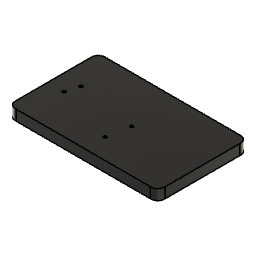
Modelo_Mesa_Optica (Autodesk Fusion 360 design; units mm, degrees)
Autodesk Fusion 360 part; units mm, degrees
sketch "Boceto1" plane through (0, 0, 0) normal (0, 0, 1) x (1, 0, 0)
  line L0 (-149.7985, 59.453) -> (50.2015, 59.453)
  line L1 (50.2015, 59.453) -> (50.2015, -60.547)
  line L2 (50.2015, -60.547) -> (-149.7985, -60.547)
  line L3 (-149.7985, -60.547) -> (-149.7985, 59.453)
  dimension "d22" = 120
  dimension "d23" = 200
  constraint horizontal L0
  constraint vertical L1
  constraint horizontal L2
  constraint vertical L3
  measures "d22" distance of L0.start L2.end
  measures "d23" distance of L1.end L2.end
extrude "Extruir1" add sketch "Boceto1" along normal blind 14
sketch "Boceto2" plane through (0, 0, 14) normal (0, 0, 1) x (-1, 0, 0)
  line L0 (20.6762, 30) -> (45, 30) construction
  line L1 (149.7985, 60.547) -> (-50.2015, 60.547)
  line L2 (-50.2015, 60.547) -> (-50.2015, -59.453)
  line L3 (-50.2015, -59.453) -> (149.7985, -59.453)
  line L4 (149.7985, -59.453) -> (149.7985, 60.547)
  point P0 (10, 22.1935)
  constraint horizontal L0
sketch "Boceto3" plane through (0, 0, 14) normal (0, 0, 1) x (-1, 0, 0)
  line L0 (149.7985, 60.547) -> (-50.2015, 60.547)
  line L1 (-50.2015, 60.547) -> (-50.2015, -59.453)
  line L2 (-50.2015, -59.453) -> (149.7985, -59.453)
  line L3 (149.7985, -59.453) -> (149.7985, 60.547)
  point P0 (42.5281, 2.6613)
  point P1 (48, 33)
  point P2 (48, 33)
  point P3 (42.5281, 2.6613)
  point P4 (48, 33)
  constraint coincident P4 P1
fillet "Empalme4" radius 10 curvature continuous 4 edges at (50.2015, -60.547, 7) (50.2015, 59.453, 7) (-149.7985, -60.547, 7) (-149.7985, 59.453, 7)
sketch "Boceto8" plane through (0, 0, 14) normal (0, 0, 1) x (-1, 0, 0)
  spline S0 degree 3 poles (149.7985, -49.453) (149.7985, -50.668) (149.7985, -51.9663) (149.0302, -54.4198) (148.4983, -55.3796) (147.0782, -57.0748) (146.1617, -57.882) (144.0991, -58.9533) (143.2175, -59.1873) (141.5243, -59.453) (140.6468, -59.453) (139.7985, -59.453) knots 0 0 0 0 0.364508 0.364508 0.64228 0.64228 0.897844 0.897844 1.107941 1.107941 1.359936 1.359936 1.359936 1.359936
  line L0 (149.7985, -49.453) -> (149.7985, 50.547)
  spline S1 degree 3 poles (139.7985, 60.547) (141.0136, 60.547) (142.3119, 60.547) (144.7654, 59.7787) (145.7252, 59.2468) (147.4204, 57.8267) (148.2276, 56.9102) (149.2989, 54.8476) (149.5329, 53.966) (149.7985, 52.2728) (149.7985, 51.3953) (149.7985, 50.547) knots 0 0 0 0 0.364508 0.364508 0.64228 0.64228 0.897844 0.897844 1.107941 1.107941 1.359936 1.359936 1.359936 1.359936
  line L1 (139.7985, 60.547) -> (-40.2015, 60.547)
  spline S2 degree 3 poles (-50.2015, 50.547) (-50.2015, 51.7621) (-50.2015, 53.0604) (-49.4331, 55.5139) (-48.9012, 56.4737) (-47.4811, 58.1689) (-46.5646, 58.9761) (-44.502, 60.0474) (-43.6204, 60.2813) (-41.9272, 60.547) (-41.0497, 60.547) (-40.2015, 60.547) knots 0 0 0 0 0.364508 0.364508 0.64228 0.64228 0.897844 0.897844 1.107941 1.107941 1.359936 1.359936 1.359936 1.359936
  line L2 (-50.2015, 50.547) -> (-50.2015, -49.453)
  spline S3 degree 3 poles (-40.2015, -59.453) (-41.4165, -59.453) (-42.7148, -59.453) (-45.1683, -58.6846) (-46.1281, -58.1528) (-47.8233, -56.7326) (-48.6305, -55.8162) (-49.7018, -53.7535) (-49.9358, -52.8719) (-50.2015, -51.1788) (-50.2015, -50.3012) (-50.2015, -49.453) knots 0 0 0 0 0.364508 0.364508 0.64228 0.64228 0.897844 0.897844 1.107941 1.107941 1.359936 1.359936 1.359936 1.359936
  line L3 (-40.2015, -59.453) -> (139.7985, -59.453)
  circle A0 centre (48, 33) radius 3
  circle A1 centre (48, 33) radius 2.25
  dimension "d52" = 4.5
  constraint concentric A0 A1
  measures "d52" diameter of A1
hole "Agujero3" at (-48, -33, 14) direction (0, 0, -1) diameter 4.5 depth 7.5 tip angle 180
thread "Rosca3" "ISO Metric profile 4.0 M4x0.7 6H" major diameter 4.1095 minor diameter 3.332 pitch 0.7 angle 60 modelled right hand crest width 0.193 on face at (-49.687, -34.4888, 11.5) crest through (-46.334, -33, 13.825)
sketch "Boceto9" plane through (0, 0, 14) normal (0, 0, 1) x (-1, 0, 0)
  circle A0 centre (122.9, -9.5) radius 3
  circle A1 centre (122.9, -9.5) radius 2.25
  dimension "d58" = 4.5
  constraint concentric A0 A1
  measures "d58" diameter of A1
hole "Agujero4" at (-122.9, 9.5, 14) direction (0, 0, -1) diameter 4.5 depth 7.5 tip angle 180
thread "Rosca4" "ISO Metric profile 4.0 M4x0.7 6H" major diameter 4.1095 minor diameter 3.332 pitch 0.7 angle 60 modelled right hand crest width 0.193 on face at (-122.026, 11.5733, 11.5) crest through (-121.234, 9.5, 13.825)
sketch "Boceto10" plane through (0, 0, 14) normal (0, 0, 1) x (-1, 0, 0)
  spline S0 degree 3 poles (123.4302, -7.5148) (123.6756, -7.6057) (123.9013, -7.7428) (124.2791, -8.0907) (124.43, -8.2953) (124.6392, -8.7429) (124.6987, -8.98) (124.7212, -9.4541) (124.6877, -9.6863) (124.5636, -10.0347) (124.5024, -10.1583) (124.3534, -10.3852) (124.267, -10.488) (124.1691, -10.5794) knots 0 0 0 0 0.078521 0.078521 0.154183 0.154183 0.226983 0.226983 0.296921 0.296921 0.338304 0.338304 0.378622 0.378622 0.378622 0.378622
  arc A0 (121.6309, -10.5794) -> (124.1691, -10.5794) centre (122.9, -9.5) ccw
  spline S1 degree 3 poles (121.6309, -10.5794) (121.4699, -10.4292) (121.3405, -10.2484) (121.1524, -9.8393) (121.0989, -9.6133) (121.0794, -9.144) (121.1171, -8.905) (121.2838, -8.445) (121.4145, -8.2298) (121.6884, -7.9279) (121.8085, -7.8241) (122.0736, -7.645) (122.2181, -7.571) (122.3698, -7.5148) knots 0 0 0 0 0.066052 0.066052 0.134957 0.134957 0.206715 0.206715 0.281323 0.281323 0.328596 0.328596 0.376941 0.376941 0.376941 0.376941
  arc A1 (123.4302, -7.5148) -> (122.3698, -7.5148) centre (122.9, -9.5) ccw
  spline S2 degree 3 poles (48.5302, 34.9852) (48.7756, 34.8943) (49.0013, 34.7572) (49.3791, 34.4093) (49.53, 34.2047) (49.7392, 33.7571) (49.7987, 33.52) (49.8212, 33.0459) (49.7877, 32.8137) (49.6636, 32.4653) (49.6024, 32.3417) (49.4534, 32.1148) (49.367, 32.012) (49.2691, 31.9206) knots 0 0 0 0 0.078521 0.078521 0.154183 0.154183 0.226983 0.226983 0.296921 0.296921 0.338304 0.338304 0.378622 0.378622 0.378622 0.378622
  arc A2 (46.7309, 31.9206) -> (49.2691, 31.9206) centre (48, 33) ccw
  spline S3 degree 3 poles (46.7309, 31.9206) (46.5699, 32.0708) (46.4405, 32.2516) (46.2524, 32.6607) (46.1989, 32.8867) (46.1794, 33.356) (46.2171, 33.595) (46.3838, 34.055) (46.5145, 34.2702) (46.7884, 34.5721) (46.9085, 34.6759) (47.1736, 34.855) (47.3181, 34.929) (47.4698, 34.9852) knots 0 0 0 0 0.066052 0.066052 0.134957 0.134957 0.206715 0.206715 0.281323 0.281323 0.328596 0.328596 0.376941 0.376941 0.376941 0.376941
  arc A3 (48.5302, 34.9852) -> (47.4698, 34.9852) centre (48, 33) ccw
  spline S4 degree 3 poles (149.7985, -49.453) (149.7985, -50.668) (149.7985, -51.9663) (149.0302, -54.4198) (148.4983, -55.3796) (147.0782, -57.0748) (146.1617, -57.882) (144.0991, -58.9533) (143.2175, -59.1873) (141.5243, -59.453) (140.6468, -59.453) (139.7985, -59.453) knots 0 0 0 0 0.364508 0.364508 0.64228 0.64228 0.897844 0.897844 1.107941 1.107941 1.359936 1.359936 1.359936 1.359936
  line L0 (149.7985, -49.453) -> (149.7985, 50.547)
  spline S5 degree 3 poles (139.7985, 60.547) (141.0136, 60.547) (142.3119, 60.547) (144.7654, 59.7787) (145.7252, 59.2468) (147.4204, 57.8267) (148.2276, 56.9102) (149.2989, 54.8476) (149.5329, 53.966) (149.7985, 52.2728) (149.7985, 51.3953) (149.7985, 50.547) knots 0 0 0 0 0.364508 0.364508 0.64228 0.64228 0.897844 0.897844 1.107941 1.107941 1.359936 1.359936 1.359936 1.359936
  line L1 (139.7985, 60.547) -> (-40.2015, 60.547)
  spline S6 degree 3 poles (-50.2015, 50.547) (-50.2015, 51.7621) (-50.2015, 53.0604) (-49.4331, 55.5139) (-48.9012, 56.4737) (-47.4811, 58.1689) (-46.5646, 58.9761) (-44.502, 60.0474) (-43.6204, 60.2813) (-41.9272, 60.547) (-41.0497, 60.547) (-40.2015, 60.547) knots 0 0 0 0 0.364508 0.364508 0.64228 0.64228 0.897844 0.897844 1.107941 1.107941 1.359936 1.359936 1.359936 1.359936
  line L2 (-50.2015, 50.547) -> (-50.2015, -49.453)
  spline S7 degree 3 poles (-40.2015, -59.453) (-41.4165, -59.453) (-42.7148, -59.453) (-45.1683, -58.6846) (-46.1281, -58.1528) (-47.8233, -56.7326) (-48.6305, -55.8162) (-49.7018, -53.7535) (-49.9358, -52.8719) (-50.2015, -51.1788) (-50.2015, -50.3012) (-50.2015, -49.453) knots 0 0 0 0 0.364508 0.364508 0.64228 0.64228 0.897844 0.897844 1.107941 1.107941 1.359936 1.359936 1.359936 1.359936
  line L3 (-40.2015, -59.453) -> (139.7985, -59.453)
  circle A4 centre (42.4509, 3) radius 3
  circle A5 centre (42.4509, 3) radius 2.25
  dimension "d64" = 4.5
  constraint concentric A4 A5
  measures "d64" diameter of A5
hole "Agujero5" at (-42.4509, -3, 14) direction (0, 0, -1) diameter 4.5 depth 7.5 tip angle 180
thread "Rosca5" "ISO Metric profile 4.0 M4x0.7 6H" major diameter 4.1095 minor diameter 3.332 pitch 0.7 angle 60 modelled right hand crest width 0.193 on face at (-42.2268, -0.7612, 11.5) crest through (-40.7849, -3, 13.825)
sketch "Boceto11" plane through (0, 0, 14) normal (0, 0, 1) x (-1, 0, 0)
  spline S0 degree 3 poles (42.981, 4.9852) (43.2265, 4.8943) (43.4522, 4.7572) (43.83, 4.4093) (43.9809, 4.2047) (44.19, 3.7571) (44.2496, 3.52) (44.2721, 3.0459) (44.2386, 2.8137) (44.1145, 2.4653) (44.0532, 2.3417) (43.9043, 2.1148) (43.8178, 2.012) (43.7199, 1.9206) knots 0 0 0 0 0.078521 0.078521 0.154183 0.154183 0.226983 0.226983 0.296921 0.296921 0.338304 0.338304 0.378622 0.378622 0.378622 0.378622
  arc A0 (41.1818, 1.9206) -> (43.7199, 1.9206) centre (42.4509, 3) ccw
  spline S1 degree 3 poles (41.1818, 1.9206) (41.0208, 2.0708) (40.8914, 2.2516) (40.7033, 2.6607) (40.6498, 2.8867) (40.6302, 3.356) (40.668, 3.595) (40.8346, 4.055) (40.9653, 4.2702) (41.2393, 4.5721) (41.3594, 4.6759) (41.6245, 4.855) (41.769, 4.929) (41.9207, 4.9852) knots 0 0 0 0 0.066052 0.066052 0.134957 0.134957 0.206715 0.206715 0.281323 0.281323 0.328596 0.328596 0.376941 0.376941 0.376941 0.376941
  arc A1 (42.981, 4.9852) -> (41.9207, 4.9852) centre (42.4509, 3) ccw
  spline S2 degree 3 poles (123.4302, -7.5148) (123.6756, -7.6057) (123.9013, -7.7428) (124.2791, -8.0907) (124.43, -8.2953) (124.6392, -8.7429) (124.6987, -8.98) (124.7212, -9.4541) (124.6877, -9.6863) (124.5636, -10.0347) (124.5024, -10.1583) (124.3534, -10.3852) (124.267, -10.488) (124.1691, -10.5794) knots 0 0 0 0 0.078521 0.078521 0.154183 0.154183 0.226983 0.226983 0.296921 0.296921 0.338304 0.338304 0.378622 0.378622 0.378622 0.378622
  arc A2 (121.6309, -10.5794) -> (124.1691, -10.5794) centre (122.9, -9.5) ccw
  spline S3 degree 3 poles (121.6309, -10.5794) (121.4699, -10.4292) (121.3405, -10.2484) (121.1524, -9.8393) (121.0989, -9.6133) (121.0794, -9.144) (121.1171, -8.905) (121.2838, -8.445) (121.4145, -8.2298) (121.6884, -7.9279) (121.8085, -7.8241) (122.0736, -7.645) (122.2181, -7.571) (122.3698, -7.5148) knots 0 0 0 0 0.066052 0.066052 0.134957 0.134957 0.206715 0.206715 0.281323 0.281323 0.328596 0.328596 0.376941 0.376941 0.376941 0.376941
  arc A3 (123.4302, -7.5148) -> (122.3698, -7.5148) centre (122.9, -9.5) ccw
  spline S4 degree 3 poles (48.5302, 34.9852) (48.7756, 34.8943) (49.0013, 34.7572) (49.3791, 34.4093) (49.53, 34.2047) (49.7392, 33.7571) (49.7987, 33.52) (49.8212, 33.0459) (49.7877, 32.8137) (49.6636, 32.4653) (49.6024, 32.3417) (49.4534, 32.1148) (49.367, 32.012) (49.2691, 31.9206) knots 0 0 0 0 0.078521 0.078521 0.154183 0.154183 0.226983 0.226983 0.296921 0.296921 0.338304 0.338304 0.378622 0.378622 0.378622 0.378622
  arc A4 (46.7309, 31.9206) -> (49.2691, 31.9206) centre (48, 33) ccw
  spline S5 degree 3 poles (46.7309, 31.9206) (46.5699, 32.0708) (46.4405, 32.2516) (46.2524, 32.6607) (46.1989, 32.8867) (46.1794, 33.356) (46.2171, 33.595) (46.3838, 34.055) (46.5145, 34.2702) (46.7884, 34.5721) (46.9085, 34.6759) (47.1736, 34.855) (47.3181, 34.929) (47.4698, 34.9852) knots 0 0 0 0 0.066052 0.066052 0.134957 0.134957 0.206715 0.206715 0.281323 0.281323 0.328596 0.328596 0.376941 0.376941 0.376941 0.376941
  arc A5 (48.5302, 34.9852) -> (47.4698, 34.9852) centre (48, 33) ccw
  spline S6 degree 3 poles (149.7985, -49.453) (149.7985, -50.668) (149.7985, -51.9663) (149.0302, -54.4198) (148.4983, -55.3796) (147.0782, -57.0748) (146.1617, -57.882) (144.0991, -58.9533) (143.2175, -59.1873) (141.5243, -59.453) (140.6468, -59.453) (139.7985, -59.453) knots 0 0 0 0 0.364508 0.364508 0.64228 0.64228 0.897844 0.897844 1.107941 1.107941 1.359936 1.359936 1.359936 1.359936
  line L0 (149.7985, -49.453) -> (149.7985, 50.547)
  spline S7 degree 3 poles (139.7985, 60.547) (141.0136, 60.547) (142.3119, 60.547) (144.7654, 59.7787) (145.7252, 59.2468) (147.4204, 57.8267) (148.2276, 56.9102) (149.2989, 54.8476) (149.5329, 53.966) (149.7985, 52.2728) (149.7985, 51.3953) (149.7985, 50.547) knots 0 0 0 0 0.364508 0.364508 0.64228 0.64228 0.897844 0.897844 1.107941 1.107941 1.359936 1.359936 1.359936 1.359936
  line L1 (139.7985, 60.547) -> (-40.2015, 60.547)
  spline S8 degree 3 poles (-50.2015, 50.547) (-50.2015, 51.7621) (-50.2015, 53.0604) (-49.4331, 55.5139) (-48.9012, 56.4737) (-47.4811, 58.1689) (-46.5646, 58.9761) (-44.502, 60.0474) (-43.6204, 60.2813) (-41.9272, 60.547) (-41.0497, 60.547) (-40.2015, 60.547) knots 0 0 0 0 0.364508 0.364508 0.64228 0.64228 0.897844 0.897844 1.107941 1.107941 1.359936 1.359936 1.359936 1.359936
  line L2 (-50.2015, 50.547) -> (-50.2015, -49.453)
  spline S9 degree 3 poles (-40.2015, -59.453) (-41.4165, -59.453) (-42.7148, -59.453) (-45.1683, -58.6846) (-46.1281, -58.1528) (-47.8233, -56.7326) (-48.6305, -55.8162) (-49.7018, -53.7535) (-49.9358, -52.8719) (-50.2015, -51.1788) (-50.2015, -50.3012) (-50.2015, -49.453) knots 0 0 0 0 0.364508 0.364508 0.64228 0.64228 0.897844 0.897844 1.107941 1.107941 1.359936 1.359936 1.359936 1.359936
  line L3 (-40.2015, -59.453) -> (139.7985, -59.453)
  circle A6 centre (128, 8) radius 3
  circle A7 centre (128, 8) radius 2.25
  dimension "d70" = 4.5
  constraint concentric A6 A7
  measures "d70" diameter of A7
hole "Agujero6" at (-128, -8, 14) direction (0, 0, -1) diameter 4.5 depth 7.5 tip angle 180
thread "Rosca6" "ISO Metric profile 4.0 M4x0.7 6H" major diameter 4.1095 minor diameter 3.332 pitch 0.7 angle 60 modelled right hand crest width 0.193 on face at (-129.8269, -6.6866, 11.5) crest through (-126.334, -8, 13.825)
named bodies: "Base"
